Autodesk Fusion 360 part; units mm, degrees
(part 3 of 21)
sketch "Schizzo1 (3)" plane through (0, 0, 3) normal (0, 0, 1) x (-1, 0, 0)
  arc A0 (-3.7907, 0.66) -> (-3.6757, 0.7388) centre (-3.7737, 0.7585) ccw
  arc A1 (-3.408, 1.5628) -> (-3.6757, 0.7388) centre (0, 0) ccw
  arc A2 (-3.408, 1.5628) -> (-3.4546, 1.6942) centre (-3.4988, 1.6045) ccw
  line L0 (-3.4546, 1.6942) -> (-4.2177, 2.0704)
  spline S0 degree 5 poles (-4.2177, 2.0704) (-4.2211, 2.0721) (-4.2279, 2.0756) (-4.238, 2.0812) (-4.251, 2.0893) (-4.2668, 2.1003) (-4.2822, 2.1119) (-4.2974, 2.1239) (-4.3125, 2.1362) (-4.3275, 2.1486) (-4.3425, 2.1612) (-4.3573, 2.1739) (-4.3719, 2.187) (-4.3864, 2.2004) (-4.4007, 2.214) (-4.4148, 2.228) (-4.4287, 2.2422) (-4.4426, 2.2567) (-4.4563, 2.2713) (-4.4699, 2.2861) (-4.4833, 2.301) (-4.4967, 2.3162) (-4.5099, 2.3315) (-4.523, 2.3471) (-4.536, 2.3628) (-4.5488, 2.3787) (-4.5616, 2.3948) (-4.5742, 2.4111) (-4.5866, 2.4275) (-4.599, 2.4441) (-4.6113, 2.4608) (-4.6234, 2.4777) (-4.6354, 2.4948) (-4.6473, 2.512) (-4.6591, 2.5293) (-4.6708, 2.5469) (-4.6823, 2.5645) (-4.6938, 2.5823) (-4.7051, 2.6003) (-4.7163, 2.6184) (-4.7274, 2.6366) (-4.7383, 2.655) (-4.7492, 2.6735) (-4.7599, 2.6921) (-4.7706, 2.7109) (-4.7811, 2.7298) (-4.7915, 2.7488) (-4.8017, 2.768) (-4.8119, 2.7873) (-4.822, 2.8067) (-4.8319, 2.8262) (-4.8417, 2.8459) (-4.8514, 2.8657) (-4.861, 2.8856) (-4.8705, 2.9056) (-4.8798, 2.9257) (-4.8891, 2.946) (-4.8982, 2.9663) (-4.9072, 2.9868) (-4.9161, 3.0074) (-4.9249, 3.0281) (-4.9335, 3.0489) (-4.9421, 3.0698) (-4.9505, 3.0909) (-4.9588, 3.112) (-4.967, 3.1333) (-4.975, 3.1546) (-4.983, 3.176) (-4.9908, 3.1976) (-4.9985, 3.2193) (-5.0061, 3.241) (-5.0121, 3.2585) (-5.0165, 3.2716) (-5.0195, 3.2804) (-5.0209, 3.2848) knots 0 0 0 0 0 0 0.01428571 0.02857143 0.04285714 0.05714286 0.07142857 0.08571429 0.1 0.11428571 0.12857143 0.14285714 0.15714286 0.17142857 0.18571429 0.2 0.21428571 0.22857143 0.24285714 0.25714286 0.27142857 0.28571429 0.3 0.31428571 0.32857143 0.34285714 0.35714286 0.37142857 0.38571429 0.4 0.41428571 0.42857143 0.44285714 0.45714286 0.47142857 0.48571429 0.5 0.51428571 0.52857143 0.54285714 0.55714286 0.57142857 0.58571429 0.6 0.61428571 0.62857143 0.64285714 0.65714286 0.67142857 0.68571429 0.7 0.71428571 0.72857143 0.74285714 0.75714286 0.77142857 0.78571429 0.8 0.81428571 0.82857143 0.84285714 0.85714286 0.87142857 0.88571429 0.9 0.91428571 0.92857143 0.94285714 0.95714286 0.97142857 0.98571429 1 1 1 1 1 1
  arc A3 (-4.6756, 3.7601) -> (-5.0209, 3.2848) centre (0, 0) ccw
  spline S1 degree 5 poles (-4.6756, 3.7601) (-4.671, 3.7601) (-4.6617, 3.76) (-4.6478, 3.7599) (-4.6294, 3.7596) (-4.6063, 3.7591) (-4.5833, 3.7584) (-4.5604, 3.7577) (-4.5376, 3.7567) (-4.5148, 3.7556) (-4.492, 3.7544) (-4.4694, 3.7531) (-4.4468, 3.7515) (-4.4242, 3.7499) (-4.4018, 3.7481) (-4.3794, 3.7461) (-4.357, 3.744) (-4.3348, 3.7418) (-4.3126, 3.7394) (-4.2905, 3.7369) (-4.2684, 3.7342) (-4.2465, 3.7314) (-4.2246, 3.7284) (-4.2028, 3.7253) (-4.181, 3.7221) (-4.1594, 3.7186) (-4.1378, 3.7151) (-4.1163, 3.7114) (-4.0949, 3.7075) (-4.0736, 3.7035) (-4.0524, 3.6994) (-4.0313, 3.6951) (-4.0102, 3.6906) (-3.9893, 3.686) (-3.9684, 3.6812) (-3.9476, 3.6763) (-3.927, 3.6713) (-3.9064, 3.666) (-3.8859, 3.6607) (-3.8656, 3.6551) (-3.8453, 3.6495) (-3.8251, 3.6436) (-3.8051, 3.6376) (-3.7852, 3.6315) (-3.7653, 3.6251) (-3.7456, 3.6187) (-3.726, 3.612) (-3.7066, 3.6052) (-3.6872, 3.5983) (-3.668, 3.5911) (-3.6488, 3.5838) (-3.6299, 3.5764) (-3.6111, 3.5687) (-3.5924, 3.5609) (-3.5738, 3.5528) (-3.5554, 3.5446) (-3.5372, 3.5363) (-3.519, 3.5278) (-3.501, 3.5191) (-3.4832, 3.5102) (-3.4656, 3.5011) (-3.4481, 3.4918) (-3.431, 3.4821) (-3.414, 3.4722) (-3.3973, 3.4621) (-3.3807, 3.4518) (-3.3643, 3.4413) (-3.3479, 3.4308) (-3.3318, 3.42) (-3.316, 3.4089) (-3.3007, 3.3973) (-3.289, 3.3874) (-3.2805, 3.3796) (-3.2751, 3.3742) (-3.2724, 3.3715) knots -1 -1 -1 -1 -1 -1 -0.98571429 -0.97142857 -0.95714286 -0.94285714 -0.92857143 -0.91428571 -0.9 -0.88571429 -0.87142857 -0.85714286 -0.84285714 -0.82857143 -0.81428571 -0.8 -0.78571429 -0.77142857 -0.75714286 -0.74285714 -0.72857143 -0.71428571 -0.7 -0.68571429 -0.67142857 -0.65714286 -0.64285714 -0.62857143 -0.61428571 -0.6 -0.58571429 -0.57142857 -0.55714286 -0.54285714 -0.52857143 -0.51428571 -0.5 -0.48571429 -0.47142857 -0.45714286 -0.44285714 -0.42857143 -0.41428571 -0.4 -0.38571429 -0.37142857 -0.35714286 -0.34285714 -0.32857143 -0.31428571 -0.3 -0.28571429 -0.27142857 -0.25714286 -0.24285714 -0.22857143 -0.21428571 -0.2 -0.18571429 -0.17142857 -0.15714286 -0.14285714 -0.12857143 -0.11428571 -0.1 -0.08571429 -0.07142857 -0.05714286 -0.04285714 -0.02857143 -0.01428571 0 0 0 0 0 0
  line L1 (-3.2724, 3.3715) -> (-2.6788, 2.762)
  arc A4 (-2.6788, 2.762) -> (-2.5394, 2.7582) centre (-2.6072, 2.8318) ccw
  arc A5 (-1.8385, 3.2675) -> (-2.5394, 2.7582) centre (0, 0) ccw
  arc A6 (-1.8385, 3.2675) -> (-1.799, 3.4012) centre (-1.8875, 3.3546) ccw
  line L2 (-1.799, 3.4012) -> (-2.1952, 4.1541)
  spline S2 degree 5 poles (-2.1952, 4.1541) (-2.197, 4.1575) (-2.2005, 4.1643) (-2.2053, 4.1748) (-2.2111, 4.189) (-2.2174, 4.2071) (-2.223, 4.2256) (-2.2283, 4.2442) (-2.2333, 4.263) (-2.2381, 4.2819) (-2.2428, 4.3008) (-2.2473, 4.3199) (-2.2515, 4.3391) (-2.2553, 4.3584) (-2.2588, 4.3779) (-2.262, 4.3974) (-2.265, 4.4171) (-2.2677, 4.4369) (-2.2702, 4.4568) (-2.2725, 4.4768) (-2.2746, 4.4968) (-2.2765, 4.5169) (-2.2782, 4.5371) (-2.2796, 4.5574) (-2.2809, 4.5777) (-2.2819, 4.5982) (-2.2828, 4.6187) (-2.2834, 4.6392) (-2.2838, 4.6598) (-2.2841, 4.6805) (-2.2842, 4.7013) (-2.284, 4.7221) (-2.2837, 4.7429) (-2.2833, 4.7639) (-2.2826, 4.7848) (-2.2817, 4.8059) (-2.2807, 4.8269) (-2.2795, 4.8481) (-2.2781, 4.8693) (-2.2765, 4.8905) (-2.2748, 4.9117) (-2.2728, 4.933) (-2.2707, 4.9544) (-2.2685, 4.9758) (-2.266, 4.9972) (-2.2634, 5.0187) (-2.2607, 5.0402) (-2.2577, 5.0618) (-2.2546, 5.0833) (-2.2513, 5.1049) (-2.2479, 5.1266) (-2.2443, 5.1483) (-2.2405, 5.17) (-2.2365, 5.1917) (-2.2324, 5.2135) (-2.2282, 5.2353) (-2.2237, 5.2571) (-2.2192, 5.2789) (-2.2144, 5.3008) (-2.2095, 5.3226) (-2.2044, 5.3446) (-2.1992, 5.3665) (-2.1938, 5.3884) (-2.1883, 5.4104) (-2.1825, 5.4324) (-2.1767, 5.4544) (-2.1707, 5.4764) (-2.1645, 5.4984) (-2.1582, 5.5204) (-2.1517, 5.5425) (-2.145, 5.5646) (-2.1396, 5.5822) (-2.1354, 5.5955) (-2.1326, 5.6043) (-2.1312, 5.6087) knots 0 0 0 0 0 0 0.01428571 0.02857143 0.04285714 0.05714286 0.07142857 0.08571429 0.1 0.11428571 0.12857143 0.14285714 0.15714286 0.17142857 0.18571429 0.2 0.21428571 0.22857143 0.24285714 0.25714286 0.27142857 0.28571429 0.3 0.31428571 0.32857143 0.34285714 0.35714286 0.37142857 0.38571429 0.4 0.41428571 0.42857143 0.44285714 0.45714286 0.47142857 0.48571429 0.5 0.51428571 0.52857143 0.54285714 0.55714286 0.57142857 0.58571429 0.6 0.61428571 0.62857143 0.64285714 0.65714286 0.67142857 0.68571429 0.7 0.71428571 0.72857143 0.74285714 0.75714286 0.77142857 0.78571429 0.8 0.81428571 0.82857143 0.84285714 0.85714286 0.87142857 0.88571429 0.9 0.91428571 0.92857143 0.94285714 0.95714286 0.97142857 0.98571429 1 1 1 1 1 1
  arc A7 (-1.5725, 5.7903) -> (-2.1312, 5.6087) centre (0, 0) ccw
  spline S3 degree 5 poles (-1.5725, 5.7903) (-1.5688, 5.7875) (-1.5613, 5.782) (-1.5502, 5.7737) (-1.5354, 5.7626) (-1.5171, 5.7487) (-1.4988, 5.7347) (-1.4808, 5.7206) (-1.4628, 5.7064) (-1.445, 5.6921) (-1.4273, 5.6778) (-1.4098, 5.6633) (-1.3924, 5.6488) (-1.3752, 5.6342) (-1.358, 5.6196) (-1.3411, 5.6048) (-1.3242, 5.59) (-1.3075, 5.5751) (-1.291, 5.5601) (-1.2746, 5.5451) (-1.2583, 5.53) (-1.2422, 5.5148) (-1.2262, 5.4995) (-1.2104, 5.4842) (-1.1948, 5.4688) (-1.1793, 5.4533) (-1.1639, 5.4377) (-1.1487, 5.4221) (-1.1337, 5.4064) (-1.1188, 5.3906) (-1.104, 5.3748) (-1.0895, 5.3589) (-1.0751, 5.3429) (-1.0608, 5.3269) (-1.0467, 5.3107) (-1.0328, 5.2946) (-1.0191, 5.2783) (-1.0055, 5.262) (-0.9921, 5.2456) (-0.9789, 5.2292) (-0.9658, 5.2127) (-0.9529, 5.1961) (-0.9402, 5.1795) (-0.9277, 5.1628) (-0.9154, 5.146) (-0.9033, 5.1292) (-0.8913, 5.1123) (-0.8796, 5.0953) (-0.868, 5.0783) (-0.8566, 5.0613) (-0.8454, 5.0441) (-0.8345, 5.0269) (-0.8238, 5.0097) (-0.8133, 4.9923) (-0.803, 4.975) (-0.7929, 4.9575) (-0.7831, 4.94) (-0.7734, 4.9225) (-0.7639, 4.9049) (-0.7547, 4.8872) (-0.7458, 4.8695) (-0.7372, 4.8517) (-0.729, 4.8338) (-0.7211, 4.8158) (-0.7135, 4.7977) (-0.7061, 4.7797) (-0.699, 4.7615) (-0.692, 4.7434) (-0.6853, 4.7252) (-0.679, 4.707) (-0.6734, 4.6886) (-0.6697, 4.6737) (-0.6675, 4.6624) (-0.6663, 4.6549) (-0.6658, 4.6511) knots -1 -1 -1 -1 -1 -1 -0.98571429 -0.97142857 -0.95714286 -0.94285714 -0.92857143 -0.91428571 -0.9 -0.88571429 -0.87142857 -0.85714286 -0.84285714 -0.82857143 -0.81428571 -0.8 -0.78571429 -0.77142857 -0.75714286 -0.74285714 -0.72857143 -0.71428571 -0.7 -0.68571429 -0.67142857 -0.65714286 -0.64285714 -0.62857143 -0.61428571 -0.6 -0.58571429 -0.57142857 -0.55714286 -0.54285714 -0.52857143 -0.51428571 -0.5 -0.48571429 -0.47142857 -0.45714286 -0.44285714 -0.42857143 -0.41428571 -0.4 -0.38571429 -0.37142857 -0.35714286 -0.34285714 -0.32857143 -0.31428571 -0.3 -0.28571429 -0.27142857 -0.25714286 -0.24285714 -0.22857143 -0.21428571 -0.2 -0.18571429 -0.17142857 -0.15714286 -0.14285714 -0.12857143 -0.11428571 -0.1 -0.08571429 -0.07142857 -0.05714286 -0.04285714 -0.02857143 -0.01428571 0 0 0 0 0 0
  line L3 (-0.6658, 4.6511) -> (-0.5437, 3.8091)
  arc A8 (-0.5437, 3.8091) -> (-0.4332, 3.7241) centre (-0.4448, 3.8234) ccw
  arc A9 (0.4332, 3.7241) -> (-0.4332, 3.7241) centre (0, 0) ccw
  arc A10 (0.4332, 3.7241) -> (0.5437, 3.8091) centre (0.4448, 3.8234) ccw
  line L4 (0.5437, 3.8091) -> (0.6658, 4.6511)
  spline S4 degree 5 poles (0.6658, 4.6511) (0.6663, 4.6549) (0.6675, 4.6624) (0.6697, 4.6737) (0.6734, 4.6886) (0.679, 4.707) (0.6853, 4.7252) (0.692, 4.7434) (0.699, 4.7615) (0.7061, 4.7797) (0.7135, 4.7977) (0.7211, 4.8158) (0.729, 4.8338) (0.7372, 4.8517) (0.7458, 4.8695) (0.7547, 4.8872) (0.7639, 4.9049) (0.7734, 4.9225) (0.7831, 4.94) (0.7929, 4.9575) (0.803, 4.975) (0.8133, 4.9923) (0.8238, 5.0097) (0.8345, 5.0269) (0.8454, 5.0441) (0.8566, 5.0613) (0.868, 5.0783) (0.8796, 5.0953) (0.8913, 5.1123) (0.9033, 5.1292) (0.9154, 5.146) (0.9277, 5.1628) (0.9402, 5.1795) (0.9529, 5.1961) (0.9658, 5.2127) (0.9789, 5.2292) (0.9921, 5.2456) (1.0055, 5.262) (1.0191, 5.2783) (1.0328, 5.2946) (1.0467, 5.3107) (1.0608, 5.3269) (1.0751, 5.3429) (1.0895, 5.3589) (1.104, 5.3748) (1.1188, 5.3906) (1.1337, 5.4064) (1.1487, 5.4221) (1.1639, 5.4377) (1.1793, 5.4533) (1.1948, 5.4688) (1.2104, 5.4842) (1.2262, 5.4995) (1.2422, 5.5148) (1.2583, 5.53) (1.2746, 5.5451) (1.291, 5.5601) (1.3075, 5.5751) (1.3242, 5.59) (1.3411, 5.6048) (1.358, 5.6196) (1.3752, 5.6342) (1.3924, 5.6488) (1.4098, 5.6633) (1.4273, 5.6778) (1.445, 5.6921) (1.4628, 5.7064) (1.4808, 5.7206) (1.4988, 5.7347) (1.5171, 5.7487) (1.5354, 5.7626) (1.5502, 5.7737) (1.5613, 5.782) (1.5688, 5.7875) (1.5725, 5.7903) knots 0 0 0 0 0 0 0.01428571 0.02857143 0.04285714 0.05714286 0.07142857 0.08571429 0.1 0.11428571 0.12857143 0.14285714 0.15714286 0.17142857 0.18571429 0.2 0.21428571 0.22857143 0.24285714 0.25714286 0.27142857 0.28571429 0.3 0.31428571 0.32857143 0.34285714 0.35714286 0.37142857 0.38571429 0.4 0.41428571 0.42857143 0.44285714 0.45714286 0.47142857 0.48571429 0.5 0.51428571 0.52857143 0.54285714 0.55714286 0.57142857 0.58571429 0.6 0.61428571 0.62857143 0.64285714 0.65714286 0.67142857 0.68571429 0.7 0.71428571 0.72857143 0.74285714 0.75714286 0.77142857 0.78571429 0.8 0.81428571 0.82857143 0.84285714 0.85714286 0.87142857 0.88571429 0.9 0.91428571 0.92857143 0.94285714 0.95714286 0.97142857 0.98571429 1 1 1 1 1 1
  arc A11 (2.1312, 5.6087) -> (1.5725, 5.7903) centre (0, 0) ccw
  spline S5 degree 5 poles (2.1312, 5.6087) (2.1326, 5.6043) (2.1354, 5.5955) (2.1396, 5.5822) (2.145, 5.5646) (2.1517, 5.5425) (2.1582, 5.5204) (2.1645, 5.4984) (2.1707, 5.4764) (2.1767, 5.4544) (2.1825, 5.4324) (2.1883, 5.4104) (2.1938, 5.3884) (2.1992, 5.3665) (2.2044, 5.3446) (2.2095, 5.3226) (2.2144, 5.3008) (2.2192, 5.2789) (2.2237, 5.2571) (2.2282, 5.2353) (2.2324, 5.2135) (2.2365, 5.1917) (2.2405, 5.17) (2.2443, 5.1483) (2.2479, 5.1266) (2.2513, 5.1049) (2.2546, 5.0833) (2.2577, 5.0618) (2.2607, 5.0402) (2.2634, 5.0187) (2.266, 4.9972) (2.2685, 4.9758) (2.2707, 4.9544) (2.2728, 4.933) (2.2748, 4.9117) (2.2765, 4.8905) (2.2781, 4.8693) (2.2795, 4.8481) (2.2807, 4.8269) (2.2817, 4.8059) (2.2826, 4.7848) (2.2833, 4.7639) (2.2837, 4.7429) (2.284, 4.7221) (2.2842, 4.7013) (2.2841, 4.6805) (2.2838, 4.6598) (2.2834, 4.6392) (2.2828, 4.6187) (2.2819, 4.5982) (2.2809, 4.5777) (2.2796, 4.5574) (2.2782, 4.5371) (2.2765, 4.5169) (2.2746, 4.4968) (2.2725, 4.4768) (2.2702, 4.4568) (2.2677, 4.4369) (2.265, 4.4171) (2.262, 4.3974) (2.2588, 4.3779) (2.2553, 4.3584) (2.2515, 4.3391) (2.2473, 4.3199) (2.2428, 4.3008) (2.2381, 4.2819) (2.2333, 4.263) (2.2283, 4.2442) (2.223, 4.2256) (2.2174, 4.2071) (2.2111, 4.189) (2.2053, 4.1748) (2.2005, 4.1643) (2.197, 4.1575) (2.1952, 4.1541) knots -1 -1 -1 -1 -1 -1 -0.98571429 -0.97142857 -0.95714286 -0.94285714 -0.92857143 -0.91428571 -0.9 -0.88571429 -0.87142857 -0.85714286 -0.84285714 -0.82857143 -0.81428571 -0.8 -0.78571429 -0.77142857 -0.75714286 -0.74285714 -0.72857143 -0.71428571 -0.7 -0.68571429 -0.67142857 -0.65714286 -0.64285714 -0.62857143 -0.61428571 -0.6 -0.58571429 -0.57142857 -0.55714286 -0.54285714 -0.52857143 -0.51428571 -0.5 -0.48571429 -0.47142857 -0.45714286 -0.44285714 -0.42857143 -0.41428571 -0.4 -0.38571429 -0.37142857 -0.35714286 -0.34285714 -0.32857143 -0.31428571 -0.3 -0.28571429 -0.27142857 -0.25714286 -0.24285714 -0.22857143 -0.21428571 -0.2 -0.18571429 -0.17142857 -0.15714286 -0.14285714 -0.12857143 -0.11428571 -0.1 -0.08571429 -0.07142857 -0.05714286 -0.04285714 -0.02857143 -0.01428571 0 0 0 0 0 0
  line L5 (2.1952, 4.1541) -> (1.799, 3.4012)
  arc A12 (1.799, 3.4012) -> (1.8385, 3.2675) centre (1.8875, 3.3546) ccw
  arc A13 (2.5394, 2.7582) -> (1.8385, 3.2675) centre (0, 0) ccw
  arc A14 (2.5394, 2.7582) -> (2.6788, 2.762) centre (2.6072, 2.8318) ccw
  line L6 (2.6788, 2.762) -> (3.2724, 3.3715)
  spline S6 degree 5 poles (3.2724, 3.3715) (3.2751, 3.3742) (3.2805, 3.3796) (3.289, 3.3874) (3.3007, 3.3973) (3.316, 3.4089) (3.3318, 3.42) (3.3479, 3.4308) (3.3643, 3.4413) (3.3807, 3.4518) (3.3973, 3.4621) (3.414, 3.4722) (3.431, 3.4821) (3.4481, 3.4918) (3.4656, 3.5011) (3.4832, 3.5102) (3.501, 3.5191) (3.519, 3.5278) (3.5372, 3.5363) (3.5554, 3.5446) (3.5738, 3.5528) (3.5924, 3.5609) (3.6111, 3.5687) (3.6299, 3.5764) (3.6488, 3.5838) (3.668, 3.5911) (3.6872, 3.5983) (3.7066, 3.6052) (3.726, 3.612) (3.7456, 3.6187) (3.7653, 3.6251) (3.7852, 3.6315) (3.8051, 3.6376) (3.8251, 3.6436) (3.8453, 3.6495) (3.8656, 3.6551) (3.8859, 3.6607) (3.9064, 3.666) (3.927, 3.6713) (3.9476, 3.6763) (3.9684, 3.6812) (3.9893, 3.686) (4.0102, 3.6906) (4.0313, 3.6951) (4.0524, 3.6994) (4.0736, 3.7035) (4.0949, 3.7075) (4.1163, 3.7114) (4.1378, 3.7151) (4.1594, 3.7186) (4.181, 3.7221) (4.2028, 3.7253) (4.2246, 3.7284) (4.2465, 3.7314) (4.2684, 3.7342) (4.2905, 3.7369) (4.3126, 3.7394) (4.3348, 3.7418) (4.357, 3.744) (4.3794, 3.7461) (4.4018, 3.7481) (4.4242, 3.7499) (4.4468, 3.7515) (4.4694, 3.7531) (4.492, 3.7544) (4.5148, 3.7556) (4.5376, 3.7567) (4.5604, 3.7577) (4.5833, 3.7584) (4.6063, 3.7591) (4.6294, 3.7596) (4.6478, 3.7599) (4.6617, 3.76) (4.671, 3.7601) (4.6756, 3.7601) knots 0 0 0 0 0 0 0.01428571 0.02857143 0.04285714 0.05714286 0.07142857 0.08571429 0.1 0.11428571 0.12857143 0.14285714 0.15714286 0.17142857 0.18571429 0.2 0.21428571 0.22857143 0.24285714 0.25714286 0.27142857 0.28571429 0.3 0.31428571 0.32857143 0.34285714 0.35714286 0.37142857 0.38571429 0.4 0.41428571 0.42857143 0.44285714 0.45714286 0.47142857 0.48571429 0.5 0.51428571 0.52857143 0.54285714 0.55714286 0.57142857 0.58571429 0.6 0.61428571 0.62857143 0.64285714 0.65714286 0.67142857 0.68571429 0.7 0.71428571 0.72857143 0.74285714 0.75714286 0.77142857 0.78571429 0.8 0.81428571 0.82857143 0.84285714 0.85714286 0.87142857 0.88571429 0.9 0.91428571 0.92857143 0.94285714 0.95714286 0.97142857 0.98571429 1 1 1 1 1 1
  arc A15 (5.0209, 3.2848) -> (4.6756, 3.7601) centre (0, 0) ccw
  spline S7 degree 5 poles (5.0209, 3.2848) (5.0195, 3.2804) (5.0165, 3.2716) (5.0121, 3.2585) (5.0061, 3.241) (4.9985, 3.2193) (4.9908, 3.1976) (4.983, 3.176) (4.975, 3.1546) (4.967, 3.1333) (4.9588, 3.112) (4.9505, 3.0909) (4.9421, 3.0698) (4.9335, 3.0489) (4.9249, 3.0281) (4.9161, 3.0074) (4.9072, 2.9868) (4.8982, 2.9663) (4.8891, 2.946) (4.8798, 2.9257) (4.8705, 2.9056) (4.861, 2.8856) (4.8514, 2.8657) (4.8417, 2.8459) (4.8319, 2.8262) (4.822, 2.8067) (4.8119, 2.7873) (4.8017, 2.768) (4.7915, 2.7488) (4.7811, 2.7298) (4.7706, 2.7109) (4.7599, 2.6921) (4.7492, 2.6735) (4.7383, 2.655) (4.7274, 2.6366) (4.7163, 2.6184) (4.7051, 2.6003) (4.6938, 2.5823) (4.6823, 2.5645) (4.6708, 2.5469) (4.6591, 2.5293) (4.6473, 2.512) (4.6354, 2.4948) (4.6234, 2.4777) (4.6113, 2.4608) (4.599, 2.4441) (4.5866, 2.4275) (4.5742, 2.4111) (4.5616, 2.3948) (4.5488, 2.3787) (4.536, 2.3628) (4.523, 2.3471) (4.5099, 2.3315) (4.4967, 2.3162) (4.4833, 2.301) (4.4699, 2.2861) (4.4563, 2.2713) (4.4426, 2.2567) (4.4287, 2.2422) (4.4148, 2.228) (4.4007, 2.214) (4.3864, 2.2004) (4.3719, 2.187) (4.3573, 2.1739) (4.3425, 2.1612) (4.3275, 2.1486) (4.3125, 2.1362) (4.2974, 2.1239) (4.2822, 2.1119) (4.2668, 2.1003) (4.251, 2.0893) (4.238, 2.0812) (4.2279, 2.0756) (4.2211, 2.0721) (4.2177, 2.0704) knots -1 -1 -1 -1 -1 -1 -0.98571429 -0.97142857 -0.95714286 -0.94285714 -0.92857143 -0.91428571 -0.9 -0.88571429 -0.87142857 -0.85714286 -0.84285714 -0.82857143 -0.81428571 -0.8 -0.78571429 -0.77142857 -0.75714286 -0.74285714 -0.72857143 -0.71428571 -0.7 -0.68571429 -0.67142857 -0.65714286 -0.64285714 -0.62857143 -0.61428571 -0.6 -0.58571429 -0.57142857 -0.55714286 -0.54285714 -0.52857143 -0.51428571 -0.5 -0.48571429 -0.47142857 -0.45714286 -0.44285714 -0.42857143 -0.41428571 -0.4 -0.38571429 -0.37142857 -0.35714286 -0.34285714 -0.32857143 -0.31428571 -0.3 -0.28571429 -0.27142857 -0.25714286 -0.24285714 -0.22857143 -0.21428571 -0.2 -0.18571429 -0.17142857 -0.15714286 -0.14285714 -0.12857143 -0.11428571 -0.1 -0.08571429 -0.07142857 -0.05714286 -0.04285714 -0.02857143 -0.01428571 0 0 0 0 0 0
  line L7 (4.2177, 2.0704) -> (3.4546, 1.6942)
  arc A16 (3.4546, 1.6942) -> (3.408, 1.5628) centre (3.4988, 1.6045) ccw
  arc A17 (3.6757, 0.7388) -> (3.408, 1.5628) centre (0, 0) ccw
  arc A18 (3.6757, 0.7388) -> (3.7907, 0.66) centre (3.7737, 0.7585) ccw
  line L8 (3.7907, 0.66) -> (4.6291, 0.8041)
  spline S8 degree 5 poles (4.6291, 0.8041) (4.6329, 0.8047) (4.6405, 0.8059) (4.6519, 0.8073) (4.6672, 0.8084) (4.6864, 0.8088) (4.7057, 0.8085) (4.7251, 0.8077) (4.7445, 0.8066) (4.7639, 0.8054) (4.7834, 0.804) (4.8029, 0.8024) (4.8224, 0.8004) (4.842, 0.7981) (4.8616, 0.7954) (4.8812, 0.7924) (4.9009, 0.7891) (4.9205, 0.7856) (4.9402, 0.7818) (4.9599, 0.7778) (4.9796, 0.7737) (4.9993, 0.7693) (5.019, 0.7646) (5.0388, 0.7598) (5.0585, 0.7547) (5.0783, 0.7493) (5.098, 0.7438) (5.1178, 0.738) (5.1375, 0.7321) (5.1573, 0.7259) (5.177, 0.7196) (5.1968, 0.7131) (5.2165, 0.7063) (5.2363, 0.6994) (5.256, 0.6923) (5.2757, 0.685) (5.2955, 0.6775) (5.3152, 0.6698) (5.3349, 0.6619) (5.3546, 0.6538) (5.3743, 0.6456) (5.394, 0.6372) (5.4136, 0.6286) (5.4333, 0.6198) (5.4529, 0.6109) (5.4725, 0.6018) (5.4921, 0.5925) (5.5117, 0.583) (5.5312, 0.5734) (5.5508, 0.5636) (5.5703, 0.5536) (5.5898, 0.5435) (5.6093, 0.5332) (5.6287, 0.5228) (5.6482, 0.5121) (5.6676, 0.5013) (5.6869, 0.4904) (5.7063, 0.4793) (5.7256, 0.468) (5.7449, 0.4566) (5.7642, 0.445) (5.7834, 0.4332) (5.8026, 0.4213) (5.8218, 0.4093) (5.8409, 0.397) (5.86, 0.3847) (5.8791, 0.3721) (5.8982, 0.3595) (5.9172, 0.3466) (5.9361, 0.3336) (5.9551, 0.3205) (5.9702, 0.3099) (5.9815, 0.3018) (5.989, 0.2964) (5.9928, 0.2937) knots 0 0 0 0 0 0 0.01428571 0.02857143 0.04285714 0.05714286 0.07142857 0.08571429 0.1 0.11428571 0.12857143 0.14285714 0.15714286 0.17142857 0.18571429 0.2 0.21428571 0.22857143 0.24285714 0.25714286 0.27142857 0.28571429 0.3 0.31428571 0.32857143 0.34285714 0.35714286 0.37142857 0.38571429 0.4 0.41428571 0.42857143 0.44285714 0.45714286 0.47142857 0.48571429 0.5 0.51428571 0.52857143 0.54285714 0.55714286 0.57142857 0.58571429 0.6 0.61428571 0.62857143 0.64285714 0.65714286 0.67142857 0.68571429 0.7 0.71428571 0.72857143 0.74285714 0.75714286 0.77142857 0.78571429 0.8 0.81428571 0.82857143 0.84285714 0.85714286 0.87142857 0.88571429 0.9 0.91428571 0.92857143 0.94285714 0.95714286 0.97142857 0.98571429 1 1 1 1 1 1
  arc A19 (5.9928, -0.2937) -> (5.9928, 0.2937) centre (0, 0) ccw
  spline S9 degree 5 poles (5.9928, -0.2937) (5.989, -0.2964) (5.9815, -0.3018) (5.9702, -0.3099) (5.9551, -0.3205) (5.9361, -0.3336) (5.9172, -0.3466) (5.8982, -0.3595) (5.8791, -0.3721) (5.86, -0.3847) (5.8409, -0.397) (5.8218, -0.4093) (5.8026, -0.4213) (5.7834, -0.4332) (5.7642, -0.445) (5.7449, -0.4566) (5.7256, -0.468) (5.7063, -0.4793) (5.6869, -0.4904) (5.6676, -0.5013) (5.6482, -0.5121) (5.6287, -0.5228) (5.6093, -0.5332) (5.5898, -0.5435) (5.5703, -0.5536) (5.5508, -0.5636) (5.5312, -0.5734) (5.5117, -0.583) (5.4921, -0.5925) (5.4725, -0.6018) (5.4529, -0.6109) (5.4333, -0.6198) (5.4136, -0.6286) (5.394, -0.6372) (5.3743, -0.6456) (5.3546, -0.6538) (5.3349, -0.6619) (5.3152, -0.6698) (5.2955, -0.6775) (5.2757, -0.685) (5.256, -0.6923) (5.2363, -0.6994) (5.2165, -0.7063) (5.1968, -0.7131) (5.177, -0.7196) (5.1573, -0.7259) (5.1375, -0.7321) (5.1178, -0.738) (5.098, -0.7438) (5.0783, -0.7493) (5.0585, -0.7547) (5.0388, -0.7598) (5.019, -0.7646) (4.9993, -0.7693) (4.9796, -0.7737) (4.9599, -0.7778) (4.9402, -0.7818) (4.9205, -0.7856) (4.9009, -0.7891) (4.8812, -0.7924) (4.8616, -0.7954) (4.842, -0.7981) (4.8224, -0.8004) (4.8029, -0.8024) (4.7834, -0.804) (4.7639, -0.8054) (4.7445, -0.8066) (4.7251, -0.8077) (4.7057, -0.8085) (4.6864, -0.8088) (4.6672, -0.8084) (4.6519, -0.8073) (4.6405, -0.8059) (4.6329, -0.8047) (4.6291, -0.8041) knots -1 -1 -1 -1 -1 -1 -0.98571429 -0.97142857 -0.95714286 -0.94285714 -0.92857143 -0.91428571 -0.9 -0.88571429 -0.87142857 -0.85714286 -0.84285714 -0.82857143 -0.81428571 -0.8 -0.78571429 -0.77142857 -0.75714286 -0.74285714 -0.72857143 -0.71428571 -0.7 -0.68571429 -0.67142857 -0.65714286 -0.64285714 -0.62857143 -0.61428571 -0.6 -0.58571429 -0.57142857 -0.55714286 -0.54285714 -0.52857143 -0.51428571 -0.5 -0.48571429 -0.47142857 -0.45714286 -0.44285714 -0.42857143 -0.41428571 -0.4 -0.38571429 -0.37142857 -0.35714286 -0.34285714 -0.32857143 -0.31428571 -0.3 -0.28571429 -0.27142857 -0.25714286 -0.24285714 -0.22857143 -0.21428571 -0.2 -0.18571429 -0.17142857 -0.15714286 -0.14285714 -0.12857143 -0.11428571 -0.1 -0.08571429 -0.07142857 -0.05714286 -0.04285714 -0.02857143 -0.01428571 0 0 0 0 0 0
  line L9 (4.6291, -0.8041) -> (3.7907, -0.66)
  arc A20 (3.7907, -0.66) -> (3.6757, -0.7388) centre (3.7737, -0.7585) ccw
  arc A21 (3.408, -1.5628) -> (3.6757, -0.7388) centre (0, 0) ccw
  arc A22 (3.408, -1.5628) -> (3.4546, -1.6942) centre (3.4988, -1.6045) ccw
  line L10 (3.4546, -1.6942) -> (4.2177, -2.0704)
  spline S10 degree 5 poles (4.2177, -2.0704) (4.2211, -2.0721) (4.2279, -2.0756) (4.238, -2.0812) (4.251, -2.0893) (4.2668, -2.1003) (4.2822, -2.1119) (4.2974, -2.1239) (4.3125, -2.1362) (4.3275, -2.1486) (4.3425, -2.1612) (4.3573, -2.1739) (4.3719, -2.187) (4.3864, -2.2004) (4.4007, -2.214) (4.4148, -2.228) (4.4287, -2.2422) (4.4426, -2.2567) (4.4563, -2.2713) (4.4699, -2.2861) (4.4833, -2.301) (4.4967, -2.3162) (4.5099, -2.3315) (4.523, -2.3471) (4.536, -2.3628) (4.5488, -2.3787) (4.5616, -2.3948) (4.5742, -2.4111) (4.5866, -2.4275) (4.599, -2.4441) (4.6113, -2.4608) (4.6234, -2.4777) (4.6354, -2.4948) (4.6473, -2.512) (4.6591, -2.5293) (4.6708, -2.5469) (4.6823, -2.5645) (4.6938, -2.5823) (4.7051, -2.6003) (4.7163, -2.6184) (4.7274, -2.6366) (4.7383, -2.655) (4.7492, -2.6735) (4.7599, -2.6921) (4.7706, -2.7109) (4.7811, -2.7298) (4.7915, -2.7488) (4.8017, -2.768) (4.8119, -2.7873) (4.822, -2.8067) (4.8319, -2.8262) (4.8417, -2.8459) (4.8514, -2.8657) (4.861, -2.8856) (4.8705, -2.9056) (4.8798, -2.9257) (4.8891, -2.946) (4.8982, -2.9663) (4.9072, -2.9868) (4.9161, -3.0074) (4.9249, -3.0281) (4.9335, -3.0489) (4.9421, -3.0698) (4.9505, -3.0909) (4.9588, -3.112) (4.967, -3.1333) (4.975, -3.1546) (4.983, -3.176) (4.9908, -3.1976) (4.9985, -3.2193) (5.0061, -3.241) (5.0121, -3.2585) (5.0165, -3.2716) (5.0195, -3.2804) (5.0209, -3.2848) knots 0 0 0 0 0 0 0.01428571 0.02857143 0.04285714 0.05714286 0.07142857 0.08571429 0.1 0.11428571 0.12857143 0.14285714 0.15714286 0.17142857 0.18571429 0.2 0.21428571 0.22857143 0.24285714 0.25714286 0.27142857 0.28571429 0.3 0.31428571 0.32857143 0.34285714 0.35714286 0.37142857 0.38571429 0.4 0.41428571 0.42857143 0.44285714 0.45714286 0.47142857 0.48571429 0.5 0.51428571 0.52857143 0.54285714 0.55714286 0.57142857 0.58571429 0.6 0.61428571 0.62857143 0.64285714 0.65714286 0.67142857 0.68571429 0.7 0.71428571 0.72857143 0.74285714 0.75714286 0.77142857 0.78571429 0.8 0.81428571 0.82857143 0.84285714 0.85714286 0.87142857 0.88571429 0.9 0.91428571 0.92857143 0.94285714 0.95714286 0.97142857 0.98571429 1 1 1 1 1 1
  arc A23 (4.6756, -3.7601) -> (5.0209, -3.2848) centre (0, 0) ccw
  spline S11 degree 5 poles (4.6756, -3.7601) (4.671, -3.7601) (4.6617, -3.76) (4.6478, -3.7599) (4.6294, -3.7596) (4.6063, -3.7591) (4.5833, -3.7584) (4.5604, -3.7577) (4.5376, -3.7567) (4.5148, -3.7556) (4.492, -3.7544) (4.4694, -3.7531) (4.4468, -3.7515) (4.4242, -3.7499) (4.4018, -3.7481) (4.3794, -3.7461) (4.357, -3.744) (4.3348, -3.7418) (4.3126, -3.7394) (4.2905, -3.7369) (4.2684, -3.7342) (4.2465, -3.7314) (4.2246, -3.7284) (4.2028, -3.7253) (4.181, -3.7221) (4.1594, -3.7186) (4.1378, -3.7151) (4.1163, -3.7114) (4.0949, -3.7075) (4.0736, -3.7035) (4.0524, -3.6994) (4.0313, -3.6951) (4.0102, -3.6906) (3.9893, -3.686) (3.9684, -3.6812) (3.9476, -3.6763) (3.927, -3.6713) (3.9064, -3.666) (3.8859, -3.6607) (3.8656, -3.6551) (3.8453, -3.6495) (3.8251, -3.6436) (3.8051, -3.6376) (3.7852, -3.6315) (3.7653, -3.6251) (3.7456, -3.6187) (3.726, -3.612) (3.7066, -3.6052) (3.6872, -3.5983) (3.668, -3.5911) (3.6488, -3.5838) (3.6299, -3.5764) (3.6111, -3.5687) (3.5924, -3.5609) (3.5738, -3.5528) (3.5554, -3.5446) (3.5372, -3.5363) (3.519, -3.5278) (3.501, -3.5191) (3.4832, -3.5102) (3.4656, -3.5011) (3.4481, -3.4918) (3.431, -3.4821) (3.414, -3.4722) (3.3973, -3.4621) (3.3807, -3.4518) (3.3643, -3.4413) (3.3479, -3.4308) (3.3318, -3.42) (3.316, -3.4089) (3.3007, -3.3973) (3.289, -3.3874) (3.2805, -3.3796) (3.2751, -3.3742) (3.2724, -3.3715) knots -1 -1 -1 -1 -1 -1 -0.98571429 -0.97142857 -0.95714286 -0.94285714 -0.92857143 -0.91428571 -0.9 -0.88571429 -0.87142857 -0.85714286 -0.84285714 -0.82857143 -0.81428571 -0.8 -0.78571429 -0.77142857 -0.75714286 -0.74285714 -0.72857143 -0.71428571 -0.7 -0.68571429 -0.67142857 -0.65714286 -0.64285714 -0.62857143 -0.61428571 -0.6 -0.58571429 -0.57142857 -0.55714286 -0.54285714 -0.52857143 -0.51428571 -0.5 -0.48571429 -0.47142857 -0.45714286 -0.44285714 -0.42857143 -0.41428571 -0.4 -0.38571429 -0.37142857 -0.35714286 -0.34285714 -0.32857143 -0.31428571 -0.3 -0.28571429 -0.27142857 -0.25714286 -0.24285714 -0.22857143 -0.21428571 -0.2 -0.18571429 -0.17142857 -0.15714286 -0.14285714 -0.12857143 -0.11428571 -0.1 -0.08571429 -0.07142857 -0.05714286 -0.04285714 -0.02857143 -0.01428571 0 0 0 0 0 0
  line L11 (3.2724, -3.3715) -> (2.6788, -2.762)
  arc A24 (2.6788, -2.762) -> (2.5394, -2.7582) centre (2.6072, -2.8318) ccw
  arc A25 (1.8385, -3.2675) -> (2.5394, -2.7582) centre (0, 0) ccw
  arc A26 (1.8385, -3.2675) -> (1.799, -3.4012) centre (1.8875, -3.3546) ccw
  line L12 (1.799, -3.4012) -> (2.1952, -4.1541)
  spline S12 degree 5 poles (2.1952, -4.1541) (2.197, -4.1575) (2.2005, -4.1643) (2.2053, -4.1748) (2.2111, -4.189) (2.2174, -4.2071) (2.223, -4.2256) (2.2283, -4.2442) (2.2333, -4.263) (2.2381, -4.2819) (2.2428, -4.3008) (2.2473, -4.3199) (2.2515, -4.3391) (2.2553, -4.3584) (2.2588, -4.3779) (2.262, -4.3974) (2.265, -4.4171) (2.2677, -4.4369) (2.2702, -4.4568) (2.2725, -4.4768) (2.2746, -4.4968) (2.2765, -4.5169) (2.2782, -4.5371) (2.2796, -4.5574) (2.2809, -4.5777) (2.2819, -4.5982) (2.2828, -4.6187) (2.2834, -4.6392) (2.2838, -4.6598) (2.2841, -4.6805) (2.2842, -4.7013) (2.284, -4.7221) (2.2837, -4.7429) (2.2833, -4.7639) (2.2826, -4.7848) (2.2817, -4.8059) (2.2807, -4.8269) (2.2795, -4.8481) (2.2781, -4.8693) (2.2765, -4.8905) (2.2748, -4.9117) (2.2728, -4.933) (2.2707, -4.9544) (2.2685, -4.9758) (2.266, -4.9972) (2.2634, -5.0187) (2.2607, -5.0402) (2.2577, -5.0618) (2.2546, -5.0833) (2.2513, -5.1049) (2.2479, -5.1266) (2.2443, -5.1483) (2.2405, -5.17) (2.2365, -5.1917) (2.2324, -5.2135) (2.2282, -5.2353) (2.2237, -5.2571) (2.2192, -5.2789) (2.2144, -5.3008) (2.2095, -5.3226) (2.2044, -5.3446) (2.1992, -5.3665) (2.1938, -5.3884) (2.1883, -5.4104) (2.1825, -5.4324) (2.1767, -5.4544) (2.1707, -5.4764) (2.1645, -5.4984) (2.1582, -5.5204) (2.1517, -5.5425) (2.145, -5.5646) (2.1396, -5.5822) (2.1354, -5.5955) (2.1326, -5.6043) (2.1312, -5.6087) knots 0 0 0 0 0 0 0.01428571 0.02857143 0.04285714 0.05714286 0.07142857 0.08571429 0.1 0.11428571 0.12857143 0.14285714 0.15714286 0.17142857 0.18571429 0.2 0.21428571 0.22857143 0.24285714 0.25714286 0.27142857 0.28571429 0.3 0.31428571 0.32857143 0.34285714 0.35714286 0.37142857 0.38571429 0.4 0.41428571 0.42857143 0.44285714 0.45714286 0.47142857 0.48571429 0.5 0.51428571 0.52857143 0.54285714 0.55714286 0.57142857 0.58571429 0.6 0.61428571 0.62857143 0.64285714 0.65714286 0.67142857 0.68571429 0.7 0.71428571 0.72857143 0.74285714 0.75714286 0.77142857 0.78571429 0.8 0.81428571 0.82857143 0.84285714 0.85714286 0.87142857 0.88571429 0.9 0.91428571 0.92857143 0.94285714 0.95714286 0.97142857 0.98571429 1 1 1 1 1 1
  arc A27 (1.5725, -5.7903) -> (2.1312, -5.6087) centre (0, 0) ccw
  spline S13 degree 5 poles (1.5725, -5.7903) (1.5688, -5.7875) (1.5613, -5.782) (1.5502, -5.7737) (1.5354, -5.7626) (1.5171, -5.7487) (1.4988, -5.7347) (1.4808, -5.7206) (1.4628, -5.7064) (1.445, -5.6921) (1.4273, -5.6778) (1.4098, -5.6633) (1.3924, -5.6488) (1.3752, -5.6342) (1.358, -5.6196) (1.3411, -5.6048) (1.3242, -5.59) (1.3075, -5.5751) (1.291, -5.5601) (1.2746, -5.5451) (1.2583, -5.53) (1.2422, -5.5148) (1.2262, -5.4995) (1.2104, -5.4842) (1.1948, -5.4688) (1.1793, -5.4533) (1.1639, -5.4377) (1.1487, -5.4221) (1.1337, -5.4064) (1.1188, -5.3906) (1.104, -5.3748) (1.0895, -5.3589) (1.0751, -5.3429) (1.0608, -5.3269) (1.0467, -5.3107) (1.0328, -5.2946) (1.0191, -5.2783) (1.0055, -5.262) (0.9921, -5.2456) (0.9789, -5.2292) (0.9658, -5.2127) (0.9529, -5.1961) (0.9402, -5.1795) (0.9277, -5.1628) (0.9154, -5.146) (0.9033, -5.1292) (0.8913, -5.1123) (0.8796, -5.0953) (0.868, -5.0783) (0.8566, -5.0613) (0.8454, -5.0441) (0.8345, -5.0269) (0.8238, -5.0097) (0.8133, -4.9923) (0.803, -4.975) (0.7929, -4.9575) (0.7831, -4.94) (0.7734, -4.9225) (0.7639, -4.9049) (0.7547, -4.8872) (0.7458, -4.8695) (0.7372, -4.8517) (0.729, -4.8338) (0.7211, -4.8158) (0.7135, -4.7977) (0.7061, -4.7797) (0.699, -4.7615) (0.692, -4.7434) (0.6853, -4.7252) (0.679, -4.707) (0.6734, -4.6886) (0.6697, -4.6737) (0.6675, -4.6624) (0.6663, -4.6549) (0.6658, -4.6511) knots -1 -1 -1 -1 -1 -1 -0.98571429 -0.97142857 -0.95714286 -0.94285714 -0.92857143 -0.91428571 -0.9 -0.88571429 -0.87142857 -0.85714286 -0.84285714 -0.82857143 -0.81428571 -0.8 -0.78571429 -0.77142857 -0.75714286 -0.74285714 -0.72857143 -0.71428571 -0.7 -0.68571429 -0.67142857 -0.65714286 -0.64285714 -0.62857143 -0.61428571 -0.6 -0.58571429 -0.57142857 -0.55714286 -0.54285714 -0.52857143 -0.51428571 -0.5 -0.48571429 -0.47142857 -0.45714286 -0.44285714 -0.42857143 -0.41428571 -0.4 -0.38571429 -0.37142857 -0.35714286 -0.34285714 -0.32857143 -0.31428571 -0.3 -0.28571429 -0.27142857 -0.25714286 -0.24285714 -0.22857143 -0.21428571 -0.2 -0.18571429 -0.17142857 -0.15714286 -0.14285714 -0.12857143 -0.11428571 -0.1 -0.08571429 -0.07142857 -0.05714286 -0.04285714 -0.02857143 -0.01428571 0 0 0 0 0 0
  line L13 (0.6658, -4.6511) -> (0.5437, -3.8091)
  arc A28 (0.5437, -3.8091) -> (0.4332, -3.7241) centre (0.4448, -3.8234) ccw
  arc A29 (-0.4332, -3.7241) -> (0.4332, -3.7241) centre (0, 0) ccw
  arc A30 (-0.4332, -3.7241) -> (-0.5437, -3.8091) centre (-0.4448, -3.8234) ccw
  line L14 (-0.5437, -3.8091) -> (-0.6658, -4.6511)
  spline S14 degree 5 poles (-0.6658, -4.6511) (-0.6663, -4.6549) (-0.6675, -4.6624) (-0.6697, -4.6737) (-0.6734, -4.6886) (-0.679, -4.707) (-0.6853, -4.7252) (-0.692, -4.7434) (-0.699, -4.7615) (-0.7061, -4.7797) (-0.7135, -4.7977) (-0.7211, -4.8158) (-0.729, -4.8338) (-0.7372, -4.8517) (-0.7458, -4.8695) (-0.7547, -4.8872) (-0.7639, -4.9049) (-0.7734, -4.9225) (-0.7831, -4.94) (-0.7929, -4.9575) (-0.803, -4.975) (-0.8133, -4.9923) (-0.8238, -5.0097) (-0.8345, -5.0269) (-0.8454, -5.0441) (-0.8566, -5.0613) (-0.868, -5.0783) (-0.8796, -5.0953) (-0.8913, -5.1123) (-0.9033, -5.1292) (-0.9154, -5.146) (-0.9277, -5.1628) (-0.9402, -5.1795) (-0.9529, -5.1961) (-0.9658, -5.2127) (-0.9789, -5.2292) (-0.9921, -5.2456) (-1.0055, -5.262) (-1.0191, -5.2783) (-1.0328, -5.2946) (-1.0467, -5.3107) (-1.0608, -5.3269) (-1.0751, -5.3429) (-1.0895, -5.3589) (-1.104, -5.3748) (-1.1188, -5.3906) (-1.1337, -5.4064) (-1.1487, -5.4221) (-1.1639, -5.4377) (-1.1793, -5.4533) (-1.1948, -5.4688) (-1.2104, -5.4842) (-1.2262, -5.4995) (-1.2422, -5.5148) (-1.2583, -5.53) (-1.2746, -5.5451) (-1.291, -5.5601) (-1.3075, -5.5751) (-1.3242, -5.59) (-1.3411, -5.6048) (-1.358, -5.6196) (-1.3752, -5.6342) (-1.3924, -5.6488) (-1.4098, -5.6633) (-1.4273, -5.6778) (-1.445, -5.6921) (-1.4628, -5.7064) (-1.4808, -5.7206) (-1.4988, -5.7347) (-1.5171, -5.7487) (-1.5354, -5.7626) (-1.5502, -5.7737) (-1.5613, -5.782) (-1.5688, -5.7875) (-1.5725, -5.7903) knots 0 0 0 0 0 0 0.01428571 0.02857143 0.04285714 0.05714286 0.07142857 0.08571429 0.1 0.11428571 0.12857143 0.14285714 0.15714286 0.17142857 0.18571429 0.2 0.21428571 0.22857143 0.24285714 0.25714286 0.27142857 0.28571429 0.3 0.31428571 0.32857143 0.34285714 0.35714286 0.37142857 0.38571429 0.4 0.41428571 0.42857143 0.44285714 0.45714286 0.47142857 0.48571429 0.5 0.51428571 0.52857143 0.54285714 0.55714286 0.57142857 0.58571429 0.6 0.61428571 0.62857143 0.64285714 0.65714286 0.67142857 0.68571429 0.7 0.71428571 0.72857143 0.74285714 0.75714286 0.77142857 0.78571429 0.8 0.81428571 0.82857143 0.84285714 0.85714286 0.87142857 0.88571429 0.9 0.91428571 0.92857143 0.94285714 0.95714286 0.97142857 0.98571429 1 1 1 1 1 1
  arc A31 (-2.1312, -5.6087) -> (-1.5725, -5.7903) centre (0, 0) ccw
  spline S15 degree 5 poles (-2.1312, -5.6087) (-2.1326, -5.6043) (-2.1354, -5.5955) (-2.1396, -5.5822) (-2.145, -5.5646) (-2.1517, -5.5425) (-2.1582, -5.5204) (-2.1645, -5.4984) (-2.1707, -5.4764) (-2.1767, -5.4544) (-2.1825, -5.4324) (-2.1883, -5.4104) (-2.1938, -5.3884) (-2.1992, -5.3665) (-2.2044, -5.3446) (-2.2095, -5.3226) (-2.2144, -5.3008) (-2.2192, -5.2789) (-2.2237, -5.2571) (-2.2282, -5.2353) (-2.2324, -5.2135) (-2.2365, -5.1917) (-2.2405, -5.17) (-2.2443, -5.1483) (-2.2479, -5.1266) (-2.2513, -5.1049) (-2.2546, -5.0833) (-2.2577, -5.0618) (-2.2607, -5.0402) (-2.2634, -5.0187) (-2.266, -4.9972) (-2.2685, -4.9758) (-2.2707, -4.9544) (-2.2728, -4.933) (-2.2748, -4.9117) (-2.2765, -4.8905) (-2.2781, -4.8693) (-2.2795, -4.8481) (-2.2807, -4.8269) (-2.2817, -4.8059) (-2.2826, -4.7848) (-2.2833, -4.7639) (-2.2837, -4.7429) (-2.284, -4.7221) (-2.2842, -4.7013) (-2.2841, -4.6805) (-2.2838, -4.6598) (-2.2834, -4.6392) (-2.2828, -4.6187) (-2.2819, -4.5982) (-2.2809, -4.5777) (-2.2796, -4.5574) (-2.2782, -4.5371) (-2.2765, -4.5169) (-2.2746, -4.4968) (-2.2725, -4.4768) (-2.2702, -4.4568) (-2.2677, -4.4369) (-2.265, -4.4171) (-2.262, -4.3974) (-2.2588, -4.3779) (-2.2553, -4.3584) (-2.2515, -4.3391) (-2.2473, -4.3199) (-2.2428, -4.3008) (-2.2381, -4.2819) (-2.2333, -4.263) (-2.2283, -4.2442) (-2.223, -4.2256) (-2.2174, -4.2071) (-2.2111, -4.189) (-2.2053, -4.1748) (-2.2005, -4.1643) (-2.197, -4.1575) (-2.1952, -4.1541) knots -1 -1 -1 -1 -1 -1 -0.98571429 -0.97142857 -0.95714286 -0.94285714 -0.92857143 -0.91428571 -0.9 -0.88571429 -0.87142857 -0.85714286 -0.84285714 -0.82857143 -0.81428571 -0.8 -0.78571429 -0.77142857 -0.75714286 -0.74285714 -0.72857143 -0.71428571 -0.7 -0.68571429 -0.67142857 -0.65714286 -0.64285714 -0.62857143 -0.61428571 -0.6 -0.58571429 -0.57142857 -0.55714286 -0.54285714 -0.52857143 -0.51428571 -0.5 -0.48571429 -0.47142857 -0.45714286 -0.44285714 -0.42857143 -0.41428571 -0.4 -0.38571429 -0.37142857 -0.35714286 -0.34285714 -0.32857143 -0.31428571 -0.3 -0.28571429 -0.27142857 -0.25714286 -0.24285714 -0.22857143 -0.21428571 -0.2 -0.18571429 -0.17142857 -0.15714286 -0.14285714 -0.12857143 -0.11428571 -0.1 -0.08571429 -0.07142857 -0.05714286 -0.04285714 -0.02857143 -0.01428571 0 0 0 0 0 0
  line L15 (-2.1952, -4.1541) -> (-1.799, -3.4012)
  arc A32 (-1.799, -3.4012) -> (-1.8385, -3.2675) centre (-1.8875, -3.3546) ccw
  arc A33 (-2.5394, -2.7582) -> (-1.8385, -3.2675) centre (0, 0) ccw
  arc A34 (-2.5394, -2.7582) -> (-2.6788, -2.762) centre (-2.6072, -2.8318) ccw
  line L16 (-2.6788, -2.762) -> (-3.2724, -3.3715)
  spline S16 degree 5 poles (-3.2724, -3.3715) (-3.2751, -3.3742) (-3.2805, -3.3796) (-3.289, -3.3874) (-3.3007, -3.3973) (-3.316, -3.4089) (-3.3318, -3.42) (-3.3479, -3.4308) (-3.3643, -3.4413) (-3.3807, -3.4518) (-3.3973, -3.4621) (-3.414, -3.4722) (-3.431, -3.4821) (-3.4481, -3.4918) (-3.4656, -3.5011) (-3.4832, -3.5102) (-3.501, -3.5191) (-3.519, -3.5278) (-3.5372, -3.5363) (-3.5554, -3.5446) (-3.5738, -3.5528) (-3.5924, -3.5609) (-3.6111, -3.5687) (-3.6299, -3.5764) (-3.6488, -3.5838) (-3.668, -3.5911) (-3.6872, -3.5983) (-3.7066, -3.6052) (-3.726, -3.612) (-3.7456, -3.6187) (-3.7653, -3.6251) (-3.7852, -3.6315) (-3.8051, -3.6376) (-3.8251, -3.6436) (-3.8453, -3.6495) (-3.8656, -3.6551) (-3.8859, -3.6607) (-3.9064, -3.666) (-3.927, -3.6713) (-3.9476, -3.6763) (-3.9684, -3.6812) (-3.9893, -3.686) (-4.0102, -3.6906) (-4.0313, -3.6951) (-4.0524, -3.6994) (-4.0736, -3.7035) (-4.0949, -3.7075) (-4.1163, -3.7114) (-4.1378, -3.7151) (-4.1594, -3.7186) (-4.181, -3.7221) (-4.2028, -3.7253) (-4.2246, -3.7284) (-4.2465, -3.7314) (-4.2684, -3.7342) (-4.2905, -3.7369) (-4.3126, -3.7394) (-4.3348, -3.7418) (-4.357, -3.744) (-4.3794, -3.7461) (-4.4018, -3.7481) (-4.4242, -3.7499) (-4.4468, -3.7515) (-4.4694, -3.7531) (-4.492, -3.7544) (-4.5148, -3.7556) (-4.5376, -3.7567) (-4.5604, -3.7577) (-4.5833, -3.7584) (-4.6063, -3.7591) (-4.6294, -3.7596) (-4.6478, -3.7599) (-4.6617, -3.76) (-4.671, -3.7601) (-4.6756, -3.7601) knots 0 0 0 0 0 0 0.01428571 0.02857143 0.04285714 0.05714286 0.07142857 0.08571429 0.1 0.11428571 0.12857143 0.14285714 0.15714286 0.17142857 0.18571429 0.2 0.21428571 0.22857143 0.24285714 0.25714286 0.27142857 0.28571429 0.3 0.31428571 0.32857143 0.34285714 0.35714286 0.37142857 0.38571429 0.4 0.41428571 0.42857143 0.44285714 0.45714286 0.47142857 0.48571429 0.5 0.51428571 0.52857143 0.54285714 0.55714286 0.57142857 0.58571429 0.6 0.61428571 0.62857143 0.64285714 0.65714286 0.67142857 0.68571429 0.7 0.71428571 0.72857143 0.74285714 0.75714286 0.77142857 0.78571429 0.8 0.81428571 0.82857143 0.84285714 0.85714286 0.87142857 0.88571429 0.9 0.91428571 0.92857143 0.94285714 0.95714286 0.97142857 0.98571429 1 1 1 1 1 1
  arc A35 (-5.0209, -3.2848) -> (-4.6756, -3.7601) centre (0, 0) ccw
  spline S17 degree 5 poles (-5.0209, -3.2848) (-5.0195, -3.2804) (-5.0165, -3.2716) (-5.0121, -3.2585) (-5.0061, -3.241) (-4.9985, -3.2193) (-4.9908, -3.1976) (-4.983, -3.176) (-4.975, -3.1546) (-4.967, -3.1333) (-4.9588, -3.112) (-4.9505, -3.0909) (-4.9421, -3.0698) (-4.9335, -3.0489) (-4.9249, -3.0281) (-4.9161, -3.0074) (-4.9072, -2.9868) (-4.8982, -2.9663) (-4.8891, -2.946) (-4.8798, -2.9257) (-4.8705, -2.9056) (-4.861, -2.8856) (-4.8514, -2.8657) (-4.8417, -2.8459) (-4.8319, -2.8262) (-4.822, -2.8067) (-4.8119, -2.7873) (-4.8017, -2.768) (-4.7915, -2.7488) (-4.7811, -2.7298) (-4.7706, -2.7109) (-4.7599, -2.6921) (-4.7492, -2.6735) (-4.7383, -2.655) (-4.7274, -2.6366) (-4.7163, -2.6184) (-4.7051, -2.6003) (-4.6938, -2.5823) (-4.6823, -2.5645) (-4.6708, -2.5469) (-4.6591, -2.5293) (-4.6473, -2.512) (-4.6354, -2.4948) (-4.6234, -2.4777) (-4.6113, -2.4608) (-4.599, -2.4441) (-4.5866, -2.4275) (-4.5742, -2.4111) (-4.5616, -2.3948) (-4.5488, -2.3787) (-4.536, -2.3628) (-4.523, -2.3471) (-4.5099, -2.3315) (-4.4967, -2.3162) (-4.4833, -2.301) (-4.4699, -2.2861) (-4.4563, -2.2713) (-4.4426, -2.2567) (-4.4287, -2.2422) (-4.4148, -2.228) (-4.4007, -2.214) (-4.3864, -2.2004) (-4.3719, -2.187) (-4.3573, -2.1739) (-4.3425, -2.1612) (-4.3275, -2.1486) (-4.3125, -2.1362) (-4.2974, -2.1239) (-4.2822, -2.1119) (-4.2668, -2.1003) (-4.251, -2.0893) (-4.238, -2.0812) (-4.2279, -2.0756) (-4.2211, -2.0721) (-4.2177, -2.0704) knots -1 -1 -1 -1 -1 -1 -0.98571429 -0.97142857 -0.95714286 -0.94285714 -0.92857143 -0.91428571 -0.9 -0.88571429 -0.87142857 -0.85714286 -0.84285714 -0.82857143 -0.81428571 -0.8 -0.78571429 -0.77142857 -0.75714286 -0.74285714 -0.72857143 -0.71428571 -0.7 -0.68571429 -0.67142857 -0.65714286 -0.64285714 -0.62857143 -0.61428571 -0.6 -0.58571429 -0.57142857 -0.55714286 -0.54285714 -0.52857143 -0.51428571 -0.5 -0.48571429 -0.47142857 -0.45714286 -0.44285714 -0.42857143 -0.41428571 -0.4 -0.38571429 -0.37142857 -0.35714286 -0.34285714 -0.32857143 -0.31428571 -0.3 -0.28571429 -0.27142857 -0.25714286 -0.24285714 -0.22857143 -0.21428571 -0.2 -0.18571429 -0.17142857 -0.15714286 -0.14285714 -0.12857143 -0.11428571 -0.1 -0.08571429 -0.07142857 -0.05714286 -0.04285714 -0.02857143 -0.01428571 0 0 0 0 0 0
  line L17 (-4.2177, -2.0704) -> (-3.4546, -1.6942)
  arc A36 (-3.4546, -1.6942) -> (-3.408, -1.5628) centre (-3.4988, -1.6045) ccw
  arc A37 (-3.6757, -0.7388) -> (-3.408, -1.5628) centre (0, 0) ccw
  arc A38 (-3.6757, -0.7388) -> (-3.7907, -0.66) centre (-3.7737, -0.7585) ccw
  line L18 (-3.7907, -0.66) -> (-4.6291, -0.8041)
  spline S18 degree 5 poles (-4.6291, -0.8041) (-4.6329, -0.8047) (-4.6405, -0.8059) (-4.6519, -0.8073) (-4.6672, -0.8084) (-4.6864, -0.8088) (-4.7057, -0.8085) (-4.7251, -0.8077) (-4.7445, -0.8066) (-4.7639, -0.8054) (-4.7834, -0.804) (-4.8029, -0.8024) (-4.8224, -0.8004) (-4.842, -0.7981) (-4.8616, -0.7954) (-4.8812, -0.7924) (-4.9009, -0.7891) (-4.9205, -0.7856) (-4.9402, -0.7818) (-4.9599, -0.7778) (-4.9796, -0.7737) (-4.9993, -0.7693) (-5.019, -0.7646) (-5.0388, -0.7598) (-5.0585, -0.7547) (-5.0783, -0.7493) (-5.098, -0.7438) (-5.1178, -0.738) (-5.1375, -0.7321) (-5.1573, -0.7259) (-5.177, -0.7196) (-5.1968, -0.7131) (-5.2165, -0.7063) (-5.2363, -0.6994) (-5.256, -0.6923) (-5.2757, -0.685) (-5.2955, -0.6775) (-5.3152, -0.6698) (-5.3349, -0.6619) (-5.3546, -0.6538) (-5.3743, -0.6456) (-5.394, -0.6372) (-5.4136, -0.6286) (-5.4333, -0.6198) (-5.4529, -0.6109) (-5.4725, -0.6018) (-5.4921, -0.5925) (-5.5117, -0.583) (-5.5312, -0.5734) (-5.5508, -0.5636) (-5.5703, -0.5536) (-5.5898, -0.5435) (-5.6093, -0.5332) (-5.6287, -0.5228) (-5.6482, -0.5121) (-5.6676, -0.5013) (-5.6869, -0.4904) (-5.7063, -0.4793) (-5.7256, -0.468) (-5.7449, -0.4566) (-5.7642, -0.445) (-5.7834, -0.4332) (-5.8026, -0.4213) (-5.8218, -0.4093) (-5.8409, -0.397) (-5.86, -0.3847) (-5.8791, -0.3721) (-5.8982, -0.3595) (-5.9172, -0.3466) (-5.9361, -0.3336) (-5.9551, -0.3205) (-5.9702, -0.3099) (-5.9815, -0.3018) (-5.989, -0.2964) (-5.9928, -0.2937) knots 0 0 0 0 0 0 0.01428571 0.02857143 0.04285714 0.05714286 0.07142857 0.08571429 0.1 0.11428571 0.12857143 0.14285714 0.15714286 0.17142857 0.18571429 0.2 0.21428571 0.22857143 0.24285714 0.25714286 0.27142857 0.28571429 0.3 0.31428571 0.32857143 0.34285714 0.35714286 0.37142857 0.38571429 0.4 0.41428571 0.42857143 0.44285714 0.45714286 0.47142857 0.48571429 0.5 0.51428571 0.52857143 0.54285714 0.55714286 0.57142857 0.58571429 0.6 0.61428571 0.62857143 0.64285714 0.65714286 0.67142857 0.68571429 0.7 0.71428571 0.72857143 0.74285714 0.75714286 0.77142857 0.78571429 0.8 0.81428571 0.82857143 0.84285714 0.85714286 0.87142857 0.88571429 0.9 0.91428571 0.92857143 0.94285714 0.95714286 0.97142857 0.98571429 1 1 1 1 1 1
  arc A39 (-5.9928, 0.2937) -> (-5.9928, -0.2937) centre (0, 0) ccw
  spline S19 degree 5 poles (-5.9928, 0.2937) (-5.989, 0.2964) (-5.9815, 0.3018) (-5.9702, 0.3099) (-5.9551, 0.3205) (-5.9361, 0.3336) (-5.9172, 0.3466) (-5.8982, 0.3595) (-5.8791, 0.3721) (-5.86, 0.3847) (-5.8409, 0.397) (-5.8218, 0.4093) (-5.8026, 0.4213) (-5.7834, 0.4332) (-5.7642, 0.445) (-5.7449, 0.4566) (-5.7256, 0.468) (-5.7063, 0.4793) (-5.6869, 0.4904) (-5.6676, 0.5013) (-5.6482, 0.5121) (-5.6287, 0.5228) (-5.6093, 0.5332) (-5.5898, 0.5435) (-5.5703, 0.5536) (-5.5508, 0.5636) (-5.5312, 0.5734) (-5.5117, 0.583) (-5.4921, 0.5925) (-5.4725, 0.6018) (-5.4529, 0.6109) (-5.4333, 0.6198) (-5.4136, 0.6286) (-5.394, 0.6372) (-5.3743, 0.6456) (-5.3546, 0.6538) (-5.3349, 0.6619) (-5.3152, 0.6698) (-5.2955, 0.6775) (-5.2757, 0.685) (-5.256, 0.6923) (-5.2363, 0.6994) (-5.2165, 0.7063) (-5.1968, 0.7131) (-5.177, 0.7196) (-5.1573, 0.7259) (-5.1375, 0.7321) (-5.1178, 0.738) (-5.098, 0.7438) (-5.0783, 0.7493) (-5.0585, 0.7547) (-5.0388, 0.7598) (-5.019, 0.7646) (-4.9993, 0.7693) (-4.9796, 0.7737) (-4.9599, 0.7778) (-4.9402, 0.7818) (-4.9205, 0.7856) (-4.9009, 0.7891) (-4.8812, 0.7924) (-4.8616, 0.7954) (-4.842, 0.7981) (-4.8224, 0.8004) (-4.8029, 0.8024) (-4.7834, 0.804) (-4.7639, 0.8054) (-4.7445, 0.8066) (-4.7251, 0.8077) (-4.7057, 0.8085) (-4.6864, 0.8088) (-4.6672, 0.8084) (-4.6519, 0.8073) (-4.6405, 0.8059) (-4.6329, 0.8047) (-4.6291, 0.8041) knots -1 -1 -1 -1 -1 -1 -0.98571429 -0.97142857 -0.95714286 -0.94285714 -0.92857143 -0.91428571 -0.9 -0.88571429 -0.87142857 -0.85714286 -0.84285714 -0.82857143 -0.81428571 -0.8 -0.78571429 -0.77142857 -0.75714286 -0.74285714 -0.72857143 -0.71428571 -0.7 -0.68571429 -0.67142857 -0.65714286 -0.64285714 -0.62857143 -0.61428571 -0.6 -0.58571429 -0.57142857 -0.55714286 -0.54285714 -0.52857143 -0.51428571 -0.5 -0.48571429 -0.47142857 -0.45714286 -0.44285714 -0.42857143 -0.41428571 -0.4 -0.38571429 -0.37142857 -0.35714286 -0.34285714 -0.32857143 -0.31428571 -0.3 -0.28571429 -0.27142857 -0.25714286 -0.24285714 -0.22857143 -0.21428571 -0.2 -0.18571429 -0.17142857 -0.15714286 -0.14285714 -0.12857143 -0.11428571 -0.1 -0.08571429 -0.07142857 -0.05714286 -0.04285714 -0.02857143 -0.01428571 0 0 0 0 0 0
  line L19 (-4.6291, 0.8041) -> (-3.7907, 0.66)
  arc A40 (-28.6914, 1.822) -> (-28.7247, 1.1871) centre (0, 0) ccw
  spline S20 degree 3 poles (-28.8074, 1.0927) (-28.7946, 1.0949) (-28.7823, 1.0996) (-28.7603, 1.1135) (-28.7507, 1.1225) (-28.7376, 1.141) (-28.7331, 1.1496) (-28.7269, 1.1679) (-28.7251, 1.1774) (-28.7247, 1.1871) knots 0 0 0 0 0.003906 0.003906 0.007813 0.007813 0.010709 0.010709 0.013605 0.013605 0.013605 0.013605
  spline S21 degree 5 poles (-28.8074, 1.0927) (-28.8098, 1.0923) (-28.8202, 1.0904) (-28.8389, 1.0871) (-28.8656, 1.0823) (-28.9005, 1.0758) (-28.9412, 1.0679) (-28.9819, 1.0597) (-29.0226, 1.0513) (-29.0633, 1.0427) (-29.104, 1.0338) (-29.1446, 1.0247) (-29.1853, 1.0153) (-29.2259, 1.0057) (-29.2665, 0.9959) (-29.3071, 0.9858) (-29.3477, 0.9755) (-29.3883, 0.965) (-29.4289, 0.9543) (-29.4694, 0.9434) (-29.5099, 0.9323) (-29.5505, 0.921) (-29.591, 0.9094) (-29.6315, 0.8977) (-29.672, 0.8858) (-29.7124, 0.8737) (-29.7529, 0.8614) (-29.7933, 0.8488) (-29.8337, 0.8361) (-29.8741, 0.8233) (-29.9145, 0.8102) (-29.9549, 0.7969) (-29.9952, 0.7835) (-30.0355, 0.7699) (-30.0759, 0.7561) (-30.1161, 0.7421) (-30.1564, 0.728) (-30.1967, 0.7137) (-30.2369, 0.6992) (-30.2771, 0.6845) (-30.3173, 0.6697) (-30.3575, 0.6547) (-30.3977, 0.6396) (-30.4378, 0.6242) (-30.4779, 0.6087) (-30.518, 0.5931) (-30.5581, 0.5773) (-30.5982, 0.5613) (-30.6382, 0.5451) (-30.6782, 0.5288) (-30.7182, 0.5124) (-30.7582, 0.4958) (-30.7981, 0.479) (-30.838, 0.4621) (-30.8779, 0.445) (-30.9178, 0.4278) (-30.9497, 0.4139) (-30.9736, 0.4034) (-30.9895, 0.3963) (-30.9975, 0.3928) knots 0.224488 0.224488 0.224488 0.224488 0.224488 0.224488 0.228571 0.242857 0.257143 0.271429 0.285714 0.3 0.314286 0.328571 0.342857 0.357143 0.371429 0.385714 0.4 0.414286 0.428571 0.442857 0.457143 0.471429 0.485714 0.5 0.514286 0.528571 0.542857 0.557143 0.571429 0.585714 0.6 0.614286 0.628571 0.642857 0.657143 0.671429 0.685714 0.7 0.714286 0.728571 0.742857 0.757143 0.771429 0.785714 0.8 0.814286 0.828571 0.842857 0.857143 0.871429 0.885714 0.9 0.914286 0.928571 0.942857 0.957143 0.971429 0.985714 1 1 1 1 1 1
  arc A41 (-30.9975, 0.3928) -> (-30.9975, -0.3928) centre (0, 0) ccw